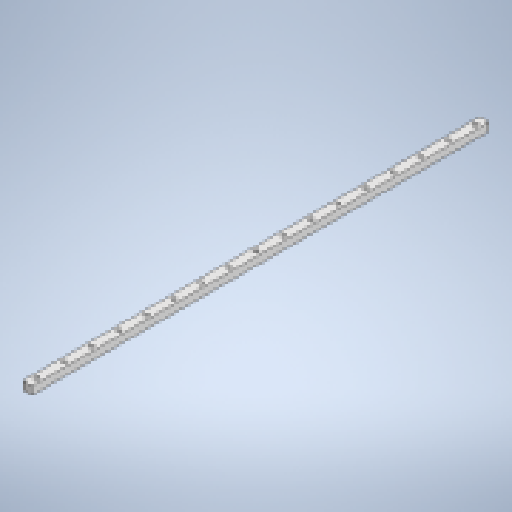
# Autodesk Inventor part: HGW20CC_Rack
Saved by Autodesk Inventor 2023 (Build 270158000, 158)
## iProperties
Created: 2022-05-01
Part Number: HGW20CC_Rack
Material: Generic
Document SubType Name: Modeling
Designer: plebbb
Density: 1 g/cm^3
Appearance: Default
Author: plebbb
Autodesk Inventor part; units mm, degrees
ref_plane "YZ Plane" through (0, 0, 0) normal (1, 0, 0) x (0, 1, 0)
ref_plane "XZ Plane" through (0, 0, 0) normal (0, 1, 0) x (-1, 0, 0)
ref_plane "XY Plane" through (0, 0, 0) normal (0, 0, 1) x (1, 0, 0)
sketch "Sketch1" plane through (0, 0, 0) normal (0, 0, 1) x (1, 0, 0)
  line L0 (0, 0) -> (20, 0)
  line L1 (20, 0) -> (20, 17.5)
  line L2 (20, 17.5) -> (0, 17.5)
  line L3 (0, 17.5) -> (0, 0)
  dimension "d0" = 20
  dimension "d1" = 17.5
  constraints: 8 end point, 2 parallel, 1 horizontal, 1 perpendicular
  measures "d0" distance of L0.start L0.end
  measures "d1" distance of L0.end L1.end
extrude "Extrusion1" add sketch "Sketch1" along normal blind 1000
sketch "Sketch2" plane through (0, 17.5, 0) normal (0, 1, 0) x (1, 0, 0)
  circle A0 centre (10, -20) radius 3
  line L0 (20, 0) -> (0, 0) projected
  point P0 (10, 0)
  dimension "d4" = 6
  dimension "d5" = 20
  constraints: 1 centre point, 1 midpoint, 1 vertical alignment
  measures "d4" diameter of A0
  measures "d5" vertical distance of L0.end A0.centre
extrude "Extrusion2" cut sketch "Sketch2" against normal up to surface (17.5 mm away)
sketch "Sketch3" plane through (0, 17.5, 0) normal (0, 1, 0) x (1, 0, 0)
  circle A0 centre (10, -20) radius 4.75
  circle A1 centre (10, -20) radius 3 construction
  point P0 (0, 0)
  dimension "d8" = 9.5
  constraints: 1 centre point, 1 concentric
  measures "d8" diameter of A0
extrude "Extrusion3" cut sketch "Sketch3" against normal blind 8.5
pattern_linear "Rectangular Pattern1" count 18 spacing 60 along (0, 0, 1) of "Extrusion2", "Extrusion3"
body "Solid1"
